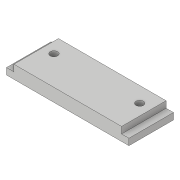
# Autodesk Inventor part: Lidar Sensor Case Piece 3
Saved by Autodesk Inventor 2018.3 (Build 223284000, 284)
## iProperties
Created: 2019-02-26
Part Number: Lidar Sensor Case Piece 3
Material: Generic
Document SubType Name: Modeling
Designer: aye06091
Mass: 5.25954 g
Surface Area: 28.8151 cm^2
Volume: 5.25954 cm^3
Density: 1 g/cm^3
Appearance: Default
Author: aye06091
Autodesk Inventor part; units mm, degrees
ref_plane "YZ Plane" through (0, 0, 0) normal (1, 0, 0) x (0, 1, 0)
ref_plane "XZ Plane" through (0, 0, 0) normal (0, 1, 0) x (-1, 0, 0)
ref_plane "XY Plane" through (0, 0, 0) normal (0, 0, 1) x (1, 0, 0)
sketch "Sketch1" plane through (0, 0, 0) normal (0, 1, 0) x (-1, 0, 0)
  line L0 (0, 0) -> (-52.8066, 0)
  line L1 (-52.8066, 0) -> (-52.8066, 19.2024)
  line L2 (-52.8066, 19.2024) -> (0, 19.2024)
  line L3 (0, 19.2024) -> (0, 0)
  dimension "d0" = 52.8066
  dimension "d1" = 19.2024
  constraints: 8 end point, 2 parallel, 1 horizontal, 1 perpendicular
  measures "d0" distance of L0.start L0.end
  measures "d1" distance of L2.end L0.start
extrude "Extrusion1" add sketch "Sketch1" along normal blind 5.6134
sketch "Sketch7" plane through (0, 5.6134, 0) normal (0, 1, 0) x (1, 0, 0)
  line L0 (0, 0) -> (0, -19.2024) projected
  line L1 (52.8066, -19.2024) -> (52.8066, 0) projected
  circle A0 centre (7.9033, -6.6524) radius 1.6
  circle A1 centre (44.9033, -6.6524) radius 1.6
  line L2 (0, -19.2024) -> (52.8066, -19.2024) projected
  dimension "d22" = 3.2
  dimension "d23" = 3.2
  dimension "d24" = 37
  dimension "d28" = 7.9033
  dimension "d29" = 7.9033
  dimension "d38" = 12.55
  constraints: 2 centre point
  measures "d22" diameter of A0
  measures "d23" diameter of A1
  measures "d24" distance of A1.centre A0.centre
  measures "d28" distance from line of L1 A1.centre
  measures "d29" distance from line of L0 A0.centre
  measures "d38" distance from line of L2 A0.centre
extrude "Extrusion6" cut sketch "Sketch7" against normal blind 25.4
sketch "Sketch8" plane through (0, 5.6134, 0) normal (0, 1, 0) x (1, 0, 0)
  line L0 (52.8066, 0) -> (0, 0) projected
  line L1 (0, 0) -> (0, -19.2024) projected
  line L2 (52.8066, -19.2024) -> (52.8066, 0) projected
  line L3 (0, -19.2024) -> (3.175, -19.2024)
  line L4 (3.175, -19.2024) -> (3.175, 0)
  line L5 (3.175, 0) -> (0, 0)
  line L6 (0, 0) -> (0, -19.2024)
  line L7 (52.8066, -19.2024) -> (49.6316, -19.2024)
  line L8 (49.6316, -19.2024) -> (49.6316, 0)
  line L9 (49.6316, 0) -> (52.8066, 0)
  line L10 (52.8066, 0) -> (52.8066, -19.2024)
  dimension "d34" = 3.175
  dimension "d35" = 3.175
  constraints: 16 end point, 4 parallel, 2 horizontal, 2 perpendicular, 2 point on line
  measures "d34" distance between parallel lines of L1 L4
  measures "d35" distance between parallel lines of L2 L8
extrude "Extrusion7" cut sketch "Sketch8" against normal blind 2.8067
equation "\"d23\" = d22"
body "Solid1"
